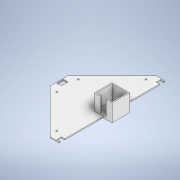
# Autodesk Inventor part: Base Definitiva
Saved by Autodesk Inventor 2021 (Build 250183000, 183)
## iProperties
Created: 2021-04-15
Part Number: Base Definitiva
Material: Plástico ABS
Document SubType Name: Modeling
Designer: Marc
Density: 1.06 g/cm^3
Appearance: Suave - Blanco
Author: Marc
Autodesk Inventor part; units mm, degrees
ref_plane "YZ Plane" through (0, 0, 0) normal (1, 0, 0) x (0, 1, 0)
ref_plane "XZ Plane" through (0, 0, 0) normal (0, 1, 0) x (-1, 0, 0)
ref_plane "XY Plane" through (0, 0, 0) normal (0, 0, 1) x (1, 0, 0)
sketch "Boceto1" plane through (0, 0, 0) normal (0, 1, 0) x (-1, 0, 0)
  line L0 (0, 145) -> (24.25, 145)
  line L1 (145, 24.25) -> (145, -24.25)
  line L2 (145, 24.25) -> (24.25, 145)
  line L3 (24.25, -145) -> (145, -24.25)
  line L4 (24.25, -145) -> (0, -145)
  circle A0 centre (29.25, -122) radius 2
  circle A1 centre (122, -29.25) radius 2
  circle A2 centre (122, 29.25) radius 2
  circle A3 centre (29.25, 122) radius 2
  line L5 (0, -145) -> (0, 145)
  point P0 (0, 0)
  dimension "d13" = 4
  dimension "d16" = 4
  dimension "d18" = 4
  dimension "d20" = 4
  constraints: 12 end point, 4 centre point, 1 horizontal
  measures "d13" diameter of A0
  measures "d16" diameter of A1
  measures "d18" diameter of A2
  measures "d20" diameter of A3
extrude "Extrusión1" add sketch "Boceto1" along normal blind 3
sketch "Boceto2" plane through (0, 3, 0) normal (0, 1, 0) x (1, 0, 0)
  line L0 (21.25, -21.25) -> (21.25, 21.25)
  line L1 (21.25, 21.25) -> (-21.25, 21.25)
  line L2 (-21.25, 21.25) -> (-21.25, -21.25)
  line L3 (-24.25, 24.25) -> (24.25, 24.25)
  line L4 (24.25, 24.25) -> (24.25, -24.25)
  line L5 (-24.25, -24.25) -> (-24.25, 24.25)
  line L6 (8.5, -21.25) -> (8.5, -24.25)
  line L7 (-8.5, -24.25) -> (-8.5, -21.25)
  line L8 (-21.25, -21.25) -> (-8.5, -21.25)
  line L9 (8.5, -21.25) -> (21.25, -21.25)
  line L10 (24.25, -24.25) -> (8.5, -24.25)
  line L11 (-8.5, -24.25) -> (-24.25, -24.25)
  dimension "d29" = 42.5
  dimension "d30" = 42.5
  dimension "d31" = 48.5
  dimension "d32" = 48.5
  constraints: 24 end point, 7 parallel, 3 horizontal, 3 perpendicular
  measures "d29" distance of L1.end L0.end
  measures "d30" distance of L0.end L0.start
  measures "d31" distance of L4.end L5.start
  measures "d32" distance of L3.end L4.end
extrude "Extrusión2" add sketch "Boceto2" along normal blind 44
sketch "Boceto3" plane through (0, 3, 0) normal (0, 1, 0) x (1, 0, 0)
  line L0 (-21.25, 21.25) -> (-21.25, -21.25) projected
  line L1 (21.25, 21.25) -> (21.25, -21.25) projected
  line L2 (-21.25, 21.25) -> (21.25, 21.25)
  line L3 (21.25, 21.25) -> (21.25, -21.25)
  line L4 (21.25, -21.25) -> (-21.25, -21.25)
  line L5 (-21.25, -21.25) -> (-21.25, 21.25)
  constraints: 8 end point, 2 parallel, 1 horizontal, 1 perpendicular
extrude "Extrusión3" add sketch "Boceto3" along normal blind 4
sketch "Boceto5" plane through (0, 3, 0) normal (0, 1, 0) x (1, 0, 0)
  line L0 (-142, 9) -> (-130, 9)
  line L1 (-130, 9) -> (-130, -9)
  line L2 (-130, -9) -> (-142, -9)
  line L3 (-9, -130) -> (-9, -142)
  line L4 (-9, 130) -> (-9, 142)
  line L5 (-142, 9) -> (-142, -9)
  line L6 (-9, -130) -> (0, -130)
  line L7 (-9, -142) -> (0, -142)
  line L8 (0, -130) -> (0, -142)
  line L9 (0, -145) -> (0, 145) projected
  line L10 (-9, 142) -> (0, 142)
  line L11 (0, 130) -> (0, 142)
  line L12 (-9, 130) -> (0, 130)
  line L13 (-8.5, -21.25) -> (-8.5, -33.25)
  line L14 (-8.5, -33.25) -> (0, -33.25)
  line L15 (0, -21.25) -> (0, -33.25)
  dimension "d72" = 12
  constraints: 30 end point, 4 perpendicular, 4 point on line, 3 collinear, 3 horizontal, 1 parallel, 1 vertical
  measures "d72" distance of L13.start L13.end
extrude "Extrusión5" cut sketch "Boceto5" against normal blind 3
sketch "Boceto8" plane through (0, 3, 0) normal (0, -1, 0) x (1, 0, 0)
  line L0 (24.25, -24.25) -> (-24.25, -24.25) projected
  line L1 (8.5, 24.25) -> (24.25, 24.25) projected
  line L2 (0, -24.25) -> (24.25, -24.25)
  line L3 (24.25, -24.25) -> (24.25, 24.25)
  line L4 (24.25, 24.25) -> (0, 24.25)
  line L5 (0, 24.25) -> (0, -24.25)
  point P0 (0, 0)
  constraints: 8 end point, 2 parallel, 1 horizontal, 1 midpoint, 1 perpendicular
extrude "Extrusión8" add sketch "Boceto8" along normal blind 3
sketch "Boceto9" plane through (-8.5, 3, 21.25) normal (0, 0, 1) x (1, 0, 0)
  line L0 (0, 0) -> (0, 4) projected
  line L1 (17, 0) -> (0, 0) projected
  line L2 (0, 4) -> (17, 4)
  line L3 (17, 4) -> (17, 0)
  line L4 (17, 0) -> (0, 0)
  line L5 (0, 0) -> (0, 4)
  point P0 (8.5, -3)
  constraints: 8 end point, 2 parallel, 1 horizontal, 1 perpendicular
extrude "Extrusión9" add sketch "Boceto9" along normal blind 3
